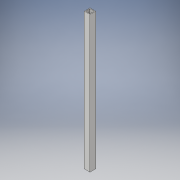
# Autodesk Inventor part: 25in 1x1 Beam
Saved by Autodesk Inventor 2018 (Build 220112000, 112)
## iProperties
Created: 2019-01-16
Part Number: 25in 1x1 Beam
Material: Generic
Document SubType Name: Modeling
Designer: Gabriel
Density: 1 g/cm^3
Appearance: Default
Author: Gabriel
Autodesk Inventor part; units mm, degrees
ref_plane "YZ Plane" through (0, 0, 0) normal (1, 0, 0) x (0, 1, 0)
ref_plane "XZ Plane" through (0, 0, 0) normal (0, 1, 0) x (-1, 0, 0)
ref_plane "XY Plane" through (0, 0, 0) normal (0, 0, 1) x (1, 0, 0)
sketch "Sketch1" plane through (0, 0, 0) normal (0, 1, 0) x (-1, 0, 0)
  line L0 (1.8436, -2.4426) -> (-23.5564, -2.4426)
  line L1 (-23.5564, -2.4426) -> (-23.5564, 22.9574)
  line L2 (-23.5564, 22.9574) -> (1.8436, 22.9574)
  line L3 (1.8436, 22.9574) -> (1.8436, -2.4426)
  line L4 (-20.3814, 0.7324) -> (-1.3314, 0.7324)
  line L5 (-1.3314, 0.7324) -> (-1.3314, 19.7824)
  line L6 (-1.3314, 19.7824) -> (-20.3814, 19.7824)
  line L7 (-20.3814, 19.7824) -> (-20.3814, 0.7324)
  point P0 (0, 0)
  dimension "d0" = 25.4
  dimension "d1" = 25.4
  dimension "d2" = 3.175
  constraints: 16 end point, 4 parallel, 2 perpendicular, 1 horizontal, 3 other
  measures "d0" distance of L1.end L2.end
  measures "d1" distance of L0.end L1.end
  measures "d2" distance between parallel lines of L0 L4
extrude "Extrusion1" add sketch "Sketch1" along normal blind 609.6
body "Solid1"
